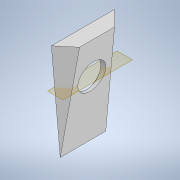
# Autodesk Inventor part: exhaustForHeater
Saved by Autodesk Inventor 2021 (Build 250183000, 183)
## iProperties
Created: 2020-07-06
Part Number: exhaustForHeater
Material: Generic
Document SubType Name: Modeling
Designer: robst
Density: 1 g/cm^3
Appearance: Default
Author: robst
Autodesk Inventor part; units mm, degrees
ref_plane "YZ Plane" through (0, 0, 0) normal (1, 0, 0) x (0, 1, 0)
ref_plane "XY Plane" through (0, 0, 0) normal (0, 0, 1) x (1, 0, 0)
sketch "Sketch1" plane through (0, 0, 0) normal (0, 0, 1) x (1, 0, 0)
  line L0 (0, 0) -> (14.2789, 101.6)
  line L1 (14.2789, 101.6) -> (0, 101.6)
  line L2 (0, 101.6) -> (0, 0)
  dimension "height" = 101.6
  dimension "d1" = 8
  dimension "d2" = 14.279
  constraints: 6 end point, 1 horizontal, 1 vertical
  measures "height" distance from line of L0.start L1
  measures "d1" angle of L0 L2
  measures "d2" distance of L0.end L1.end
extrude "MainStructure" add sketch "Sketch1" along normal mid plane 63.5
sketch "Sketch2" plane through (0, 0, 31.75) normal (-1, 0, 0) x (0, 0, 1)
  circle A0 centre (-31.75, 63.5) radius 13.97
  line L0 (-63.5, 101.6) -> (0, 101.6) projected
  line L1 (-31.75, 101.6) -> (-31.75, 0) construction
  dimension "hole" = 27.94
  dimension "centerOfHoleFromTop" = 38.1
  dimension "d29" = 0
  constraints: 2 end point, 1 centre point, 1 midpoint, 1 vertical
  measures "hole" diameter of A0
  measures "centerOfHoleFromTop" distance from line of A0.centre L0
  measures "d29" distance from line of A0.centre L1
extrude "PipeHole" cut sketch "Sketch2" against normal through all
sketch "Sketch6" plane through (0, 0, 0) normal (0, 0, 1) x (1, 0, 0)
  line L0 (0, 101.6) -> (14.2789, 101.6) projected
  line L1 (0, 0) -> (0, 101.6) projected
  line L2 (14.2789, 101.6) -> (0, 0) projected
  line L3 (0, 101.6) -> (14.1055, 100.3659)
  line L4 (14.1055, 100.3659) -> (14.2789, 101.6)
  line L5 (14.2789, 101.6) -> (0, 101.6)
  dimension "mainAngle" = 5
  constraints: 6 end point, 1 collinear, 1 point on line
  measures "mainAngle" angle of L3 L0
extrude "AngleForTopRelief" cut sketch "Sketch6" along normal through all both and the other way through all contours L0 L2 L3
sketch "Sketch7" plane through (0, 0, -31.75) normal (-1, 0, 0) x (0, 0, 1)
  line L0 (0, 0) -> (0, 101.6) construction
  line L1 (0, 38.1) -> (63.5, 38.1) construction
  line L2 (63.5, 0) -> (63.5, 100.3659) construction
  line L3 (0, 0) -> (63.5, 0) projected
  spline S0 degree 2 poles (13.5213, 31.6018) (12.7124, 31.6018) (11.3724, 32.0958) (10.8907, 32.596) knots 0 0 0 1 2 2 2
  spline S1 degree 2 poles (10.8907, 32.596) (10.4091, 33.1023) (9.8965, 34.5967) (9.8965, 35.5662) knots 0 0 0 1 2 2 2
  spline S2 degree 2 poles (9.8965, 35.5662) (9.8965, 36.4863) (10.4152, 37.9436) (10.8969, 38.4623) knots 0 0 0 1 2 2 2
  spline S3 degree 2 poles (10.8969, 38.4623) (11.36, 38.9624) (12.7185, 39.5059) (13.5275, 39.5059) knots 0 0 0 1 2 2 2
  spline S4 degree 2 poles (13.5275, 39.5059) (13.9165, 39.5059) (14.6204, 39.3947) (14.9415, 39.2959) knots 0 0 0 1 2 2 2
  spline S5 degree 2 poles (14.9415, 39.2959) (15.2009, 39.2218) (15.8307, 38.9501) (16.0222, 38.8513) knots 0 0 0 1 2 2 2
  line L4 (16.0222, 38.8513) -> (16.0222, 37.6286)
  line L5 (16.0222, 37.6286) -> (15.9357, 37.6286)
  spline S6 degree 2 poles (15.9357, 37.6286) (15.7443, 37.7954) (15.3429, 38.0979) (14.9724, 38.2708) knots 0 0 0 1 2 2 2
  spline S7 degree 2 poles (14.9724, 38.2708) (14.6637, 38.4252) (13.8671, 38.629) (13.4101, 38.629) knots 0 0 0 1 2 2 2
  spline S8 degree 2 poles (13.4101, 38.629) (12.311, 38.629) (10.9525, 36.9741) (10.9525, 35.5971) knots 0 0 0 1 2 2 2
  spline S9 degree 2 poles (10.9525, 35.5971) (10.9525, 34.8313) (11.3106, 33.6828) (11.6502, 33.2876) knots 0 0 0 1 2 2 2
  spline S10 degree 2 poles (11.6502, 33.2876) (11.9775, 32.8924) (12.9038, 32.4787) (13.4842, 32.4787) knots 0 0 0 1 2 2 2
  spline S11 degree 2 poles (13.4842, 32.4787) (13.9103, 32.4787) (14.7625, 32.6022) (15.0527, 32.7257) knots 0 0 0 1 2 2 2
  line L6 (15.0527, 32.7257) -> (15.0527, 34.6955)
  line L7 (15.0527, 34.6955) -> (13.2866, 34.6955)
  line L8 (13.2866, 34.6955) -> (13.2866, 35.5847)
  line L9 (13.2866, 35.5847) -> (16.053, 35.5847)
  line L10 (16.053, 35.5847) -> (16.053, 32.2564)
  spline S12 degree 2 poles (16.053, 32.2564) (15.8616, 32.1699) (15.2071, 31.9044) (14.9292, 31.8241) knots 0 0 0 1 2 2 2
  spline S13 degree 2 poles (14.9292, 31.8241) (14.5525, 31.7129) (13.9474, 31.6018) (13.5213, 31.6018) knots 0 0 0 1 2 2 2
  line L11 (16.5038, 31.75) -> (19.0726, 39.37)
  line L12 (19.0726, 39.37) -> (20.32, 39.37)
  line L13 (20.32, 39.37) -> (22.8888, 31.75)
  line L14 (22.8888, 31.75) -> (21.8205, 31.75)
  line L15 (21.8205, 31.75) -> (21.1289, 33.8804)
  line L16 (21.1289, 33.8804) -> (18.2205, 33.8804)
  line L17 (18.2205, 33.8804) -> (17.5289, 31.75)
  line L18 (17.5289, 31.75) -> (16.5038, 31.75)
  line L19 (20.8511, 34.7449) -> (19.6716, 38.3326)
  line L20 (19.6716, 38.3326) -> (18.4984, 34.7449)
  line L21 (18.4984, 34.7449) -> (20.8511, 34.7449)
  spline S14 degree 2 poles (25.8343, 31.6141) (25.0069, 31.6141) (23.8459, 31.96) (23.3334, 32.207) knots 0 0 0 1 2 2 2
  line L22 (23.3334, 32.207) -> (23.3334, 33.479)
  line L23 (23.3334, 33.479) -> (23.4075, 33.479)
  spline S15 degree 2 poles (23.4075, 33.479) (23.9077, 33.0097) (25.1736, 32.491) (25.7602, 32.491) knots 0 0 0 1 2 2 2
  spline S16 degree 2 poles (25.7602, 32.491) (26.6, 32.491) (27.4583, 33.1888) (27.4583, 33.7631) knots 0 0 0 1 2 2 2
  spline S17 degree 2 poles (27.4583, 33.7631) (27.4583, 34.22) (27.0076, 34.7881) (26.5197, 34.9301) knots 0 0 0 1 2 2 2
  spline S18 degree 2 poles (26.5197, 34.9301) (26.1678, 35.0289) (25.5811, 35.1648) (25.1427, 35.2759) knots 0 0 0 1 2 2 2
  spline S19 degree 2 poles (25.1427, 35.2759) (24.7475, 35.3809) (24.1238, 35.6959) (23.883, 35.949) knots 0 0 0 1 2 2 2
  spline S20 degree 2 poles (23.883, 35.949) (23.6483, 36.2022) (23.389, 36.8815) (23.389, 37.3261) knots 0 0 0 1 2 2 2
  spline S21 degree 2 poles (23.389, 37.3261) (23.389, 38.2523) (24.834, 39.5059) (25.9516, 39.5059) knots 0 0 0 1 2 2 2
  spline S22 degree 2 poles (25.9516, 39.5059) (26.5938, 39.5059) (27.73, 39.2527) (28.2179, 39.0118) knots 0 0 0 1 2 2 2
  line L24 (28.2179, 39.0118) -> (28.2179, 37.8015)
  line L25 (28.2179, 37.8015) -> (28.1438, 37.8015)
  spline S23 degree 2 poles (28.1438, 37.8015) (27.7794, 38.135) (26.6432, 38.629) (26.0196, 38.629) knots 0 0 0 1 2 2 2
  spline S24 degree 2 poles (26.0196, 38.629) (25.3156, 38.629) (24.4449, 37.9683) (24.4449, 37.431) knots 0 0 0 1 2 2 2
  spline S25 degree 2 poles (24.4449, 37.431) (24.4449, 36.9494) (24.9575, 36.3751) (25.4391, 36.2454) knots 0 0 0 1 2 2 2
  spline S26 degree 2 poles (25.4391, 36.2454) (25.7602, 36.159) (26.6926, 35.9367) (27.0014, 35.8441) knots 0 0 0 1 2 2 2
  spline S27 degree 2 poles (27.0014, 35.8441) (27.7856, 35.6032) (28.5143, 34.6337) (28.5143, 33.9236) knots 0 0 0 1 2 2 2
  spline S28 degree 2 poles (28.5143, 33.9236) (28.5143, 33.4728) (28.15, 32.6083) (27.8227, 32.3058) knots 0 0 0 1 2 2 2
  spline S29 degree 2 poles (27.8227, 32.3058) (27.4583, 31.9723) (26.5321, 31.6141) (25.8343, 31.6141) knots 0 0 0 1 2 2 2
  line L26 (37.2334, 31.75) -> (32.8183, 31.75)
  line L27 (32.8183, 31.75) -> (32.8183, 39.37)
  line L28 (32.8183, 39.37) -> (33.831, 39.37)
  line L29 (33.831, 39.37) -> (33.831, 32.6516)
  line L30 (33.831, 32.6516) -> (37.2334, 32.6516)
  line L31 (37.2334, 32.6516) -> (37.2334, 31.75)
  line L32 (40.6853, 31.75) -> (37.7336, 31.75)
  line L33 (37.7336, 31.75) -> (37.7336, 32.5281)
  line L34 (37.7336, 32.5281) -> (38.7031, 32.5281)
  line L35 (38.7031, 32.5281) -> (38.7031, 38.5919)
  line L36 (38.7031, 38.5919) -> (37.7336, 38.5919)
  line L37 (37.7336, 38.5919) -> (37.7336, 39.37)
  line L38 (37.7336, 39.37) -> (40.6853, 39.37)
  line L39 (40.6853, 39.37) -> (40.6853, 38.5919)
  line L40 (40.6853, 38.5919) -> (39.7158, 38.5919)
  line L41 (39.7158, 38.5919) -> (39.7158, 32.5281)
  line L42 (39.7158, 32.5281) -> (40.6853, 32.5281)
  line L43 (40.6853, 32.5281) -> (40.6853, 31.75)
  line L44 (47.3914, 31.75) -> (46.2552, 31.75)
  line L45 (46.2552, 31.75) -> (42.8836, 38.3202)
  line L46 (42.8836, 38.3202) -> (42.8836, 31.75)
  line L47 (42.8836, 31.75) -> (41.9388, 31.75)
  line L48 (41.9388, 31.75) -> (41.9388, 39.37)
  line L49 (41.9388, 39.37) -> (43.3776, 39.37)
  line L50 (43.3776, 39.37) -> (46.4466, 33.337)
  line L51 (46.4466, 33.337) -> (46.4466, 39.37)
  line L52 (46.4466, 39.37) -> (47.3914, 39.37)
  line L53 (47.3914, 39.37) -> (47.3914, 31.75)
  line L54 (48.9351, 31.75) -> (48.9351, 39.37)
  line L55 (48.9351, 39.37) -> (53.7023, 39.37)
  line L56 (53.7023, 39.37) -> (53.7023, 38.4684)
  line L57 (53.7023, 38.4684) -> (49.9478, 38.4684)
  line L58 (49.9478, 38.4684) -> (49.9478, 36.3813)
  line L59 (49.9478, 36.3813) -> (53.4491, 36.3813)
  line L60 (53.4491, 36.3813) -> (53.4491, 35.4797)
  line L61 (53.4491, 35.4797) -> (49.9478, 35.4797)
  line L62 (49.9478, 35.4797) -> (49.9478, 32.6516)
  line L63 (49.9478, 32.6516) -> (53.7023, 32.6516)
  line L64 (53.7023, 32.6516) -> (53.7023, 31.75)
  line L65 (53.7023, 31.75) -> (48.9351, 31.75)
  point P0 (31.75, 0)
  dimension "lineForText" = 38.1
  constraints: 2 end point, 2 horizontal, 2 point on line
  measures "lineForText" distance between parallel lines of L3 L1
extrude "TextForBack" cut sketch "Sketch7" against normal blind 1.905
sketch "Sketch8" plane through (0, 0, -31.75) normal (-1, 0, 0) x (0, 0, 1)
  circle A0 centre (31.75, 63.5) radius 13.97 projected
  circle A1 centre (31.75, 63.5) radius 19.05
  point P0 (31.75, 0)
  dimension "reliefHoleDiameter" = 38.1
  constraints: 1 centre point, 1 coincident
  measures "reliefHoleDiameter" diameter of A1
extrude "ReliefForHole" cut sketch "Sketch8" against normal blind 3.81 contours A0 | A1
sketch "Sketch9" plane through (0, 0, -31.75) normal (-1, 0, 0) x (0, 0, 1)
  line L0 (0, 100.3659) -> (0, 0) projected
  line L1 (0, 92.075) -> (63.5, 92.075) construction
  line L2 (63.5, 0) -> (63.5, 100.3659) projected
  line L3 (0, 101.6) -> (63.5, 101.6) construction
  spline S0 degree 2 poles (8.9641, 87.1272) (7.9529, 87.1272) (6.278, 87.7448) (5.6759, 88.37) knots 0 0 0 1 2 2 2
  spline S1 degree 2 poles (5.6759, 88.37) (5.0738, 89.0029) (4.4332, 90.8709) (4.4332, 92.0827) knots 0 0 0 1 2 2 2
  spline S2 degree 2 poles (4.4332, 92.0827) (4.4332, 93.2328) (5.0815, 95.0545) (5.6836, 95.7028) knots 0 0 0 1 2 2 2
  spline S3 degree 2 poles (5.6836, 95.7028) (6.2625, 96.3281) (7.9607, 97.0073) (8.9718, 97.0073) knots 0 0 0 1 2 2 2
  spline S4 degree 2 poles (8.9718, 97.0073) (9.4581, 97.0073) (10.338, 96.8684) (10.7394, 96.7449) knots 0 0 0 1 2 2 2
  spline S5 degree 2 poles (10.7394, 96.7449) (11.0636, 96.6522) (11.8509, 96.3126) (12.0902, 96.1891) knots 0 0 0 1 2 2 2
  line L4 (12.0902, 96.1891) -> (12.0902, 94.6608)
  line L5 (12.0902, 94.6608) -> (11.9822, 94.6608)
  spline S6 degree 2 poles (11.9822, 94.6608) (11.7429, 94.8692) (11.2411, 95.2474) (10.778, 95.4636) knots 0 0 0 1 2 2 2
  spline S7 degree 2 poles (10.778, 95.4636) (10.3921, 95.6565) (9.3964, 95.9112) (8.8252, 95.9112) knots 0 0 0 1 2 2 2
  spline S8 degree 2 poles (8.8252, 95.9112) (7.4512, 95.9112) (5.7531, 93.8426) (5.7531, 92.1213) knots 0 0 0 1 2 2 2
  spline S9 degree 2 poles (5.7531, 92.1213) (5.7531, 91.1642) (6.2008, 89.7285) (6.6253, 89.2345) knots 0 0 0 1 2 2 2
  spline S10 degree 2 poles (6.6253, 89.2345) (7.0344, 88.7405) (8.1922, 88.2233) (8.9178, 88.2233) knots 0 0 0 1 2 2 2
  spline S11 degree 2 poles (8.9178, 88.2233) (9.4504, 88.2233) (10.5156, 88.3777) (10.8784, 88.5321) knots 0 0 0 1 2 2 2
  line L6 (10.8784, 88.5321) -> (10.8784, 90.9944)
  line L7 (10.8784, 90.9944) -> (8.6708, 90.9944)
  line L8 (8.6708, 90.9944) -> (8.6708, 92.1059)
  line L9 (8.6708, 92.1059) -> (12.1288, 92.1059)
  line L10 (12.1288, 92.1059) -> (12.1288, 87.9454)
  spline S12 degree 2 poles (12.1288, 87.9454) (11.8895, 87.8374) (11.0713, 87.5055) (10.724, 87.4051) knots 0 0 0 1 2 2 2
  spline S13 degree 2 poles (10.724, 87.4051) (10.2531, 87.2662) (9.4967, 87.1272) (8.9641, 87.1272) knots 0 0 0 1 2 2 2
  line L11 (12.6923, 87.3125) -> (15.9033, 96.8375)
  line L12 (15.9033, 96.8375) -> (17.4625, 96.8375)
  line L13 (17.4625, 96.8375) -> (20.6735, 87.3125)
  line L14 (20.6735, 87.3125) -> (19.3382, 87.3125)
  line L15 (19.3382, 87.3125) -> (18.4737, 89.9755)
  line L16 (18.4737, 89.9755) -> (14.8381, 89.9755)
  line L17 (14.8381, 89.9755) -> (13.9736, 87.3125)
  line L18 (13.9736, 87.3125) -> (12.6923, 87.3125)
  line L19 (18.1263, 91.0561) -> (16.652, 95.5407)
  line L20 (16.652, 95.5407) -> (15.1855, 91.0561)
  line L21 (15.1855, 91.0561) -> (18.1263, 91.0561)
  spline S14 degree 2 poles (24.3554, 87.1427) (23.3211, 87.1427) (21.8699, 87.5749) (21.2293, 87.8837) knots 0 0 0 1 2 2 2
  line L22 (21.2293, 87.8837) -> (21.2293, 89.4738)
  line L23 (21.2293, 89.4738) -> (21.3219, 89.4738)
  spline S15 degree 2 poles (21.3219, 89.4738) (21.9471, 88.8871) (23.5295, 88.2388) (24.2628, 88.2388) knots 0 0 0 1 2 2 2
  spline S16 degree 2 poles (24.2628, 88.2388) (25.3125, 88.2388) (26.3854, 89.111) (26.3854, 89.8288) knots 0 0 0 1 2 2 2
  spline S17 degree 2 poles (26.3854, 89.8288) (26.3854, 90.4) (25.822, 91.1101) (25.2122, 91.2877) knots 0 0 0 1 2 2 2
  spline S18 degree 2 poles (25.2122, 91.2877) (24.7722, 91.4112) (24.0389, 91.581) (23.4909, 91.7199) knots 0 0 0 1 2 2 2
  spline S19 degree 2 poles (23.4909, 91.7199) (22.9969, 91.8512) (22.2173, 92.2448) (21.9162, 92.5613) knots 0 0 0 1 2 2 2
  spline S20 degree 2 poles (21.9162, 92.5613) (21.6229, 92.8778) (21.2987, 93.7268) (21.2987, 94.2826) knots 0 0 0 1 2 2 2
  spline S21 degree 2 poles (21.2987, 94.2826) (21.2987, 95.4404) (23.1049, 97.0073) (24.502, 97.0073) knots 0 0 0 1 2 2 2
  spline S22 degree 2 poles (24.502, 97.0073) (25.3048, 97.0073) (26.7251, 96.6908) (27.3348, 96.3898) knots 0 0 0 1 2 2 2
  line L24 (27.3348, 96.3898) -> (27.3348, 94.8769)
  line L25 (27.3348, 94.8769) -> (27.2422, 94.8769)
  spline S23 degree 2 poles (27.2422, 94.8769) (26.7868, 95.2937) (25.3666, 95.9112) (24.587, 95.9112) knots 0 0 0 1 2 2 2
  spline S24 degree 2 poles (24.587, 95.9112) (23.707, 95.9112) (22.6187, 95.0853) (22.6187, 94.4138) knots 0 0 0 1 2 2 2
  spline S25 degree 2 poles (22.6187, 94.4138) (22.6187, 93.8117) (23.2593, 93.0939) (23.8614, 92.9318) knots 0 0 0 1 2 2 2
  spline S26 degree 2 poles (23.8614, 92.9318) (24.2628, 92.8237) (25.4283, 92.5458) (25.8142, 92.4301) knots 0 0 0 1 2 2 2
  spline S27 degree 2 poles (25.8142, 92.4301) (26.7945, 92.129) (27.7053, 90.9172) (27.7053, 90.0295) knots 0 0 0 1 2 2 2
  spline S28 degree 2 poles (27.7053, 90.0295) (27.7053, 89.466) (27.2499, 88.3854) (26.8408, 88.0072) knots 0 0 0 1 2 2 2
  spline S29 degree 2 poles (26.8408, 88.0072) (26.3854, 87.5904) (25.2276, 87.1427) (24.3554, 87.1427) knots 0 0 0 1 2 2 2
  line L26 (38.6043, 87.3125) -> (33.0854, 87.3125)
  line L27 (33.0854, 87.3125) -> (33.0854, 96.8375)
  line L28 (33.0854, 96.8375) -> (34.3512, 96.8375)
  line L29 (34.3512, 96.8375) -> (34.3512, 88.4394)
  line L30 (34.3512, 88.4394) -> (38.6043, 88.4394)
  line L31 (38.6043, 88.4394) -> (38.6043, 87.3125)
  line L32 (42.9191, 87.3125) -> (39.2295, 87.3125)
  line L33 (39.2295, 87.3125) -> (39.2295, 88.2851)
  line L34 (39.2295, 88.2851) -> (40.4414, 88.2851)
  line L35 (40.4414, 88.2851) -> (40.4414, 95.8649)
  line L36 (40.4414, 95.8649) -> (39.2295, 95.8649)
  line L37 (39.2295, 95.8649) -> (39.2295, 96.8375)
  line L38 (39.2295, 96.8375) -> (42.9191, 96.8375)
  line L39 (42.9191, 96.8375) -> (42.9191, 95.8649)
  line L40 (42.9191, 95.8649) -> (41.7073, 95.8649)
  line L41 (41.7073, 95.8649) -> (41.7073, 88.2851)
  line L42 (41.7073, 88.2851) -> (42.9191, 88.2851)
  line L43 (42.9191, 88.2851) -> (42.9191, 87.3125)
  line L44 (51.3017, 87.3125) -> (49.8815, 87.3125)
  line L45 (49.8815, 87.3125) -> (45.667, 95.5253)
  line L46 (45.667, 95.5253) -> (45.667, 87.3125)
  line L47 (45.667, 87.3125) -> (44.486, 87.3125)
  line L48 (44.486, 87.3125) -> (44.486, 96.8375)
  line L49 (44.486, 96.8375) -> (46.2845, 96.8375)
  line L50 (46.2845, 96.8375) -> (50.1207, 89.2962)
  line L51 (50.1207, 89.2962) -> (50.1207, 96.8375)
  line L52 (50.1207, 96.8375) -> (51.3017, 96.8375)
  line L53 (51.3017, 96.8375) -> (51.3017, 87.3125)
  line L54 (53.2314, 87.3125) -> (53.2314, 96.8375)
  line L55 (53.2314, 96.8375) -> (59.1903, 96.8375)
  line L56 (59.1903, 96.8375) -> (59.1903, 95.7106)
  line L57 (59.1903, 95.7106) -> (54.4973, 95.7106)
  line L58 (54.4973, 95.7106) -> (54.4973, 93.1016)
  line L59 (54.4973, 93.1016) -> (58.8739, 93.1016)
  line L60 (58.8739, 93.1016) -> (58.8739, 91.9747)
  line L61 (58.8739, 91.9747) -> (54.4973, 91.9747)
  line L62 (54.4973, 91.9747) -> (54.4973, 88.4394)
  line L63 (54.4973, 88.4394) -> (59.1903, 88.4394)
  line L64 (59.1903, 88.4394) -> (59.1903, 87.3125)
  line L65 (59.1903, 87.3125) -> (53.2314, 87.3125)
  point P0 (31.75, 0)
  dimension "d35" = 9.525
  constraints: 2 end point, 2 horizontal, 2 point on line
  measures "d35" distance between parallel lines of L1 L3
extrude "TextForSmallText" cut sketch "Sketch9" against normal blind 2.54
ref_plane "Work Plane1" through (0, 101.6, 31.75) normal (0, 1, 0) x (-1, 0, 0)
sketch "Sketch10" plane through (14.1055, 100.3659, 31.75) normal (0.0871557, 0.9961947, 0) x (0.9961947, -0.0871557, 0)
  line L0 (-14.1594, 63.5) -> (-14.1594, 0) projected
  line L1 (0, 0) -> (-14.1594, 0) projected
  line L2 (0, 63.5) -> (0, 0) projected
  line L3 (-14.1594, 0) -> (0, 14.1594)
  line L4 (-14.1594, 0) -> (5.865, 0) construction
  line L5 (0, 14.1594) -> (0, 0)
  line L6 (0, 0) -> (-14.1594, 0)
  line L7 (-14.1594, 63.5) -> (0, 63.5) projected
  line L8 (-14.1594, 63.5) -> (0, 49.3406)
  line L9 (-14.1594, 63.5) -> (5.865, 63.5) construction
  line L10 (0, 49.3406) -> (0, 63.5)
  line L11 (0, 63.5) -> (-14.1594, 63.5)
  point P0 (-5.3044, 31.75)
  dimension "d38" = 45
  dimension "d39" = 45
  constraints: 16 end point, 2 collinear, 2 equal length, 2 horizontal, 2 point on line
  measures "d38" angle of L4 L3
  measures "d39" angle of L8 L9
extrude "SideAngle" cut sketch "Sketch10" against normal through all contours L7 L2 L8 | L3 L2 L1
ref_plane "Work Plane2" through (0, 63.5, 0) normal (0, 1, 0) x (-1, 0, 0)
equation "\"d42\" = height - centerOfHoleFromTop"
body "Solid1"
